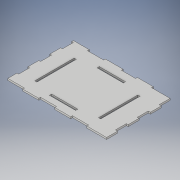
# Autodesk Inventor part: BLKG
Saved by Autodesk Inventor 2019 (Build 230136000, 136)
## iProperties
Created: 2019-11-24
Part Number: BLKG
Material: Generic
Document SubType Name: Modeling
Designer: User
Density: 1 g/cm^3
Appearance: Default
Author: User
Autodesk Inventor part; units mm, degrees
ref_plane "YZ Plane" through (0, 0, 0) normal (1, 0, 0) x (0, 1, 0)
ref_plane "XZ Plane" through (0, 0, 0) normal (0, 1, 0) x (-1, 0, 0)
ref_plane "XY Plane" through (0, 0, 0) normal (0, 0, 1) x (1, 0, 0)
sketch "Sketch1" plane through (0, 0, 0) normal (0, 1, 0) x (-1, 0, 0)
  point P0 (0, 0)
sketch "Sketch2" plane through (0, 0, 0) normal (0, 1, 0) x (-1, 0, 0)
  line L0 (55.6, -39.5) -> (55.6, -37.5)
  line L1 (55.6, -39.5) -> (37.3, -39.5)
  line L2 (37.3, -39.5) -> (37.3, -37.5)
  line L3 (37.3, -37.5) -> (19, -37.5)
  line L4 (19, -37.5) -> (19, -39.5)
  line L5 (19, -39.5) -> (0.7, -39.5)
  line L6 (-1.34, -37.5) -> (-17.6, -37.5)
  line L7 (-17.6, -37.5) -> (-17.6, -39.5)
  line L8 (-17.6, -39.5) -> (-35.9, -39.5)
  line L9 (-35.9, -39.5) -> (-35.9, -37.5)
  line L10 (-35.9, -37.5) -> (-53, -37.5)
  line L11 (-55, 37.5) -> (-36.7, 37.5)
  line L12 (-18.4, 37.5) -> (-0.1, 37.5)
  line L13 (18.2, 37.5) -> (36.5, 37.5)
  line L14 (55.6, 35.5) -> (55.6, 25)
  line L15 (55.6, 12.5) -> (55.6, 0)
  line L16 (55.6, -12.5) -> (55.6, -25)
  line L17 (55.6, 25) -> (53.6, 25)
  line L18 (53.6, 25) -> (53.6, 12.5)
  line L19 (53.6, 12.5) -> (55.6, 12.5)
  line L20 (55.6, 0) -> (53.6, 0)
  line L21 (53.6, 0) -> (53.6, -12.5)
  line L22 (53.6, -12.5) -> (55.6, -12.5)
  line L23 (55.6, -25) -> (53.6, -25)
  line L24 (53.6, -25) -> (53.6, -37.5)
  line L25 (53.6, -37.5) -> (55.6, -37.5)
  line L26 (36.5, 37.5) -> (36.5, 35.5)
  line L27 (36.5, 35.5) -> (55.6, 35.5)
  line L28 (18.2, 37.5) -> (18.2, 35.5)
  line L29 (18.2, 35.5) -> (-0.1, 35.5)
  line L30 (-0.1, 35.5) -> (-0.1, 37.5)
  line L31 (-18.4, 37.5) -> (-18.4, 35.5)
  line L32 (-18.4, 35.5) -> (-36.7, 35.5)
  line L33 (-36.7, 35.5) -> (-36.7, 37.5)
  line L34 (37.75, -22.5) -> (35.25, -22.5)
  line L35 (35.25, -22.5) -> (35.25, 22.5)
  line L36 (35.25, 22.5) -> (37.75, 22.5)
  line L37 (37.75, 22.5) -> (37.75, -22.5)
  line L38 (37.75, -22.5) -> (35.25, 22.5) construction
  line L39 (35.25, -22.5) -> (37.75, 22.5) construction
  line L40 (-37.75, -22.5) -> (-35.25, -22.5)
  line L41 (-35.25, -22.5) -> (-35.25, 22.5)
  line L42 (-35.25, 22.5) -> (-37.75, 22.5)
  line L43 (-37.75, 22.5) -> (-37.75, -22.5)
  line L44 (-37.75, -22.5) -> (-35.25, 22.5) construction
  line L45 (-35.25, -22.5) -> (-37.75, 22.5) construction
  line L46 (15, -28.4801) -> (-15, -28.4801)
  line L47 (-15, -28.4801) -> (-15, -25.9801)
  line L48 (-15, -25.9801) -> (15, -25.9801)
  line L49 (15, -25.9801) -> (15, -28.4801)
  line L50 (15, -28.4801) -> (-15, -25.9801) construction
  line L51 (-15, -28.4801) -> (15, -25.9801) construction
  line L52 (15, 28.4801) -> (-15, 28.4801)
  line L53 (-15, 28.4801) -> (-15, 25.9801)
  line L54 (-15, 25.9801) -> (15, 25.9801)
  line L55 (15, 25.9801) -> (15, 28.4801)
  line L56 (15, 28.4801) -> (-15, 25.9801) construction
  line L57 (-15, 28.4801) -> (15, 25.9801) construction
  line L58 (-53, -37.5) -> (-55, -37.5)
  line L59 (-57, -22.5) -> (-57, -22.4801)
  line L60 (-57, 37.5) -> (-55, 37.5)
  line L61 (-55, -37.5) -> (-57, -37.5)
  line L62 (-57, -37.5) -> (-57, -25)
  line L63 (-57, -25) -> (-59.4283, -25)
  line L64 (-59.4283, -25) -> (-59.4283, -12.5)
  line L65 (-59.4283, -12.5) -> (-57, -12.5)
  line L66 (-57, 0) -> (-57, -12.5)
  line L67 (-57, 0) -> (-59, 0)
  line L68 (-59, 0) -> (-59, 12.5)
  line L69 (-59, 12.5) -> (-57, 12.5)
  line L70 (-57, 12.5) -> (-57, 25)
  line L71 (-57, 25) -> (-59.4283, 25)
  line L72 (-59.4283, 25) -> (-59.4283, 37.5)
  line L73 (-59.4283, 37.5) -> (-57, 37.5)
  line L74 (0.7, -39.5) -> (-1.34, -39.5)
  line L75 (-1.34, -39.5) -> (-1.34, -37.5)
  point P0 (0.7, -37.5)
  point P1 (-55, 22.5)
  point P2 (-53, 22.5)
  point P3 (-53, 0)
  point P4 (-53, -12.5)
  point P5 (36.5, 0)
  point P6 (-36.5, 0)
  point P7 (0, -27.2301)
  point P8 (0, 27.2301)
  dimension "d55" = 18.3
  dimension "d56" = 2.04
  constraints: 152 end point, 29 point on line, 22 perpendicular, 8 horizontal, 8 midpoint, 6 parallel, 4 vertical
  measures "d55" distance of L4.end L5.end
  measures "d56" distance of L5.end L74.end
extrude "Extrusion1" add sketch "Sketch2" along normal blind 2
body "Solid1"
